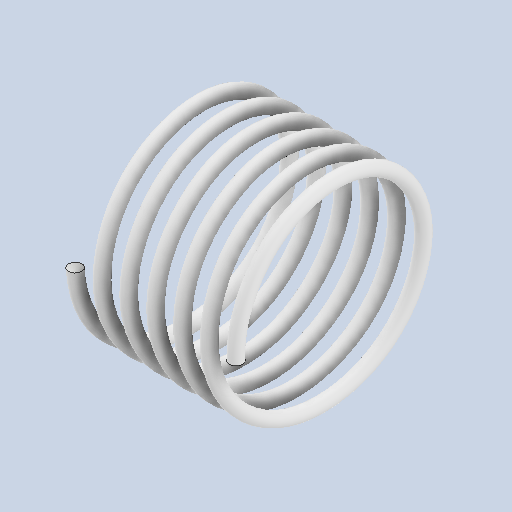
# Autodesk Inventor part: Spring_thumb
Saved by Autodesk Inventor 2022 (Build 260153000, 153)
## iProperties
Created: 2023-01-17
Part Number: Spring_thumb
Material: ABS Plastic
Document SubType Name: Modeling
Designer: 48735
Density: 1.06 g/cm^3
Appearance: Smooth - White
Author: 48735
Autodesk Inventor part; units mm, degrees
ref_plane "YZ Plane" through (0, 0, 0) normal (1, 0, 0) x (0, 1, 0)
ref_plane "XZ Plane" through (0, 0, 0) normal (0, 1, 0) x (-1, 0, 0)
ref_plane "XY Plane" through (0, 0, 0) normal (0, 0, 1) x (1, 0, 0)
sketch "Sketch1" plane through (0, 0, 0) normal (0, 1, 0) x (-1, 0, 0)
  line L0 (0, 0) -> (-3, 0)
  circle A0 centre (-3, 1.875) radius 0.125
  constraints: 2 end point, 1 centre point, 1 horizontal
coil "Coil1" sketch "Sketch1" operation add axis through (0, 0, 0) along (-1, 0, 0) pitch 0.5 turns 6 hand right
sketch "Sketch2" plane through (0, 0, 0) normal (1, 0, 0) x (0, 1, 0)
  circle A0 centre (0, 0) radius 2
  dimension "d11" = 4
  constraints: 1 centre point, 1 coincident
  measures "d11" diameter of A0
body "Solid1"
